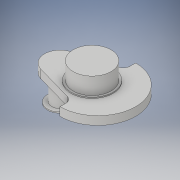
# Autodesk Inventor part: new_cigueñal
Saved by Autodesk Inventor 2019.3 (Build 233278000, 278)
## iProperties
Created: 2019-06-27
Part Number: new_cigueñal
Material: Generic
Document SubType Name: Modeling
Designer: Usuario
Density: 1 g/cm^3
Appearance: Default
Author: Usuario
Autodesk Inventor part; units mm, degrees
ref_plane "YZ Plane" through (0, 0, 0) normal (1, 0, 0) x (0, 1, 0)
ref_plane "XZ Plane" through (0, 0, 0) normal (0, 1, 0) x (-1, 0, 0)
ref_plane "XY Plane" through (0, 0, 0) normal (0, 0, 1) x (1, 0, 0)
sketch "Sketch2" plane through (0, 0, 0) normal (0, 1, 0) x (-1, 0, 0)
  circle A0 centre (0, 0) radius 28.575
  dimension "d0" = 57.15
  constraints: 1 centre point, 1 coincident
  measures "d0" diameter of A0
extrude "Extrusion1" add sketch "Sketch2" against normal blind 25.4
sketch "Sketch3" plane through (0, -25.4, 0) normal (0, -1, 0) x (1, 0, 0)
  circle A0 centre (0, 0) radius 31.75
  dimension "d3" = 63.5
  constraints: 1 centre point, 1 coincident
  measures "d3" diameter of A0
extrude "Extrusion2" add sketch "Sketch3" along normal blind 1.5875
sketch "Sketch4" plane through (0, -26.9875, 0) normal (0, -1, 0) x (1, 0, 0)
  arc A0 (8.89, -56.9095) -> (8.89, 57.3905) centre (8.89, 0.2405) ccw
  arc A1 (-54.665, 22.7287) -> (-54.665, -22.7287) centre (-48.2595, 0) ccw
  line L0 (8.89, -56.9095) -> (8.89, 57.3905) construction
  line L1 (39.6046, -49.064) -> (38.37, -48.7192)
  line L2 (8.89, -40.64) -> (-54.665, -22.7287)
  line L3 (0, 0) -> (66.0395, 0) construction
  line L4 (8.89, 40.64) -> (-54.665, 22.7287)
  line L5 (8.89, 40.64) -> (8.89, 57.3905)
  line L6 (8.89, -40.64) -> (8.89, -56.9095)
  circle A2 centre (0, 0) radius 28.575
  point P0 (-61.1412, -20.9035)
  point P1 (-61.1412, 20.9035)
  dimension "d6" = 114.3
  dimension "d7" = 47.2281
  dimension "d8" = 57.15
  dimension "d11" = 81.28
  constraints: 14 end point, 6 point on circle, 3 centre point, 3 tangent, 2 symmetric about line, 1 coincident, 1 collinear, 1 horizontal, 1 point on line, 1 vertical
  measures "d6" diameter of A0
  measures "d7" diameter of A1
  measures "d8" distance of A1.centre A0.centre
  measures "d11" distance of L4.start L2.start
extrude "Extrusion3" add sketch "Sketch4" along normal blind 12.7
fillet "Fillet1" radius 9.906 1 edges at (8.89, -33.3375, 40.64)
fillet "Fillet2" radius 9.906 1 edges at (8.89, -33.3375, -40.64)
sketch "Sketch5" plane through (0, -39.6875, 0) normal (0, -1, 0) x (1, 0, 0)
  circle A0 centre (0, 0) radius 28.575 construction
  line L0 (0, 0) -> (-72.4662, 0) construction
  circle A1 centre (-48.2595, 0) radius 19.05
  arc A2 (-54.665, 22.7287) -> (-54.665, -22.7287) centre (-48.2595, 0) ccw projected
  circle A3 centre (-48.2595, 0) radius 12.7
  point P0 (0, 0)
  dimension "d21" = 25.4
  constraints: 2 centre point, 2 end point, 1 coincident, 1 concentric, 1 horizontal, 1 point on line
  measures "d21" diameter of A3
extrude "Extrusion4" add sketch "Sketch5" along normal blind 1.5875
sketch "Sketch6" plane through (-48.2595, -39.6875, 0) normal (0, -1, 0) x (1, 0, 0)
  circle A0 centre (0, 0) radius 12.7 projected
  circle A1 centre (0, 0) radius 12.7
  point P0 (48.2595, 0)
  constraints: 1 centre point, 1 coincident
extrude "Extrusion5" cut sketch "Sketch6" against normal through all
sketch "Sketch7" plane through (0, -26.9875, 0) normal (0, 1, 0) x (1, 0, 0)
  circle A0 centre (-48.2595, 0) radius 12.7 projected
  circle A1 centre (-48.2595, 0) radius 12.7
  point P0 (0, 0)
  constraints: 1 centre point, 1 coincident
extrude "Extrusion6" add sketch "Sketch7" against normal blind 50.8
sketch "Sketch8" plane through (-48.2595, -77.7875, 0) normal (0, -1, 0) x (1, 0, 0)
  circle A0 centre (0, 0) radius 19.05
  point P0 (48.2595, 0)
  constraints: 1 centre point
extrude "Extrusion7" add sketch "Sketch8" along normal blind 1.5875
sketch "Sketch9" plane through (-48.2595, -79.375, 0) normal (0, -1, 0) x (1, 0, 0)
  point P0 (48.2595, 0)
body "Solid1"
